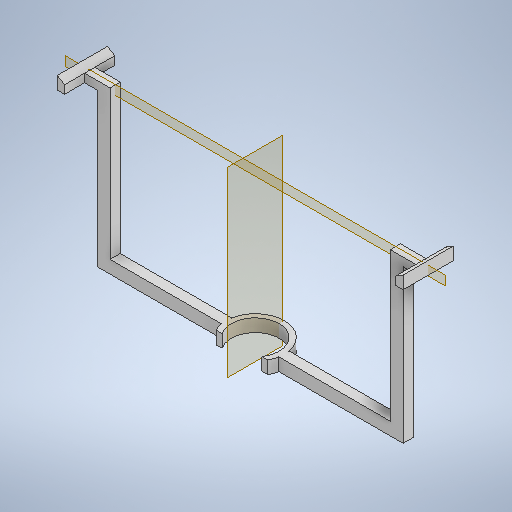
# Autodesk Inventor part: 2025_07_28_Holder_H2_O2_reactor_BOLA_GL14_V0.3
Saved by Autodesk Inventor 2025.1 (Build 291241000, 241)
## iProperties
Created: 2024-08-23
Part Number: 2025_07_28_Holder_H2_O2_reactor_BOLA_GL14_V0.3
Material: Generisch
Document SubType Name: Modeling
Designer: to86hug
Density: 1 g/cm^3
Appearance: Vorgabe
Author: to86hug
Autodesk Inventor part; units mm, degrees
ref_plane "YZ Plane" through (0, 0, 0) normal (1, 0, 0) x (0, 1, 0)
ref_plane "XZ Plane" through (0, 0, 0) normal (0, 1, 0) x (-1, 0, 0)
ref_plane "XY Plane" through (0, 0, 0) normal (0, 0, 1) x (1, 0, 0)
sketch "Skizze1" plane through (0, 0, 0) normal (0, 0, 1) x (1, 0, 0)
  line L0 (-68.016, 1.808) -> (67.584, 1.808)
  line L1 (67.584, 1.808) -> (67.584, -2.192)
  line L2 (67.584, -2.192) -> (-68.016, -2.192)
  line L3 (-68.016, -2.192) -> (-68.016, 1.808)
  line L4 (-68.016, 1.808) -> (67.584, -2.192) construction
  line L5 (67.584, 1.808) -> (-68.016, -2.192) construction
  point P0 (0, 0)
  point P1 (-0.216, -0.192)
  point P2 (-0.216, -0.192)
  dimension "d0" = 135.6
  dimension "d1" = 4
  constraints: 12 end point, 2 midpoint, 2 parallel, 1 horizontal, 1 perpendicular
  measures "d0" distance of L0.start L0.end
  measures "d1" distance of L0.end L1.end
extrude "Extrusion1" add sketch "Skizze1" along normal mid plane 3.25
ref_plane "Arbeitsebene1" through (-68.016, -0.192, 1.625) normal (0, -1, 0) x (1, 0, 0)
sketch "Skizze2" plane through (-68.016, -0.192, 1.625) normal (0, -1, 0) x (1, 0, 0)
  line L0 (0, -3.25) -> (0, 0) projected
  line L1 (0, -3.25) -> (135.6, -3.25) projected
  line L2 (0, 0) -> (2.85, 0)
  line L3 (2.85, 0) -> (2.85, -3.25)
  line L4 (2.85, -3.25) -> (0, -3.25)
  line L5 (0, -3.25) -> (0, 0)
  line L6 (0, 0) -> (0, 1.75)
  line L7 (0, 1.75) -> (2.85, 0)
  line L8 (135.6, -3.25) -> (135.6, 0) projected
  line L9 (135.6, 0) -> (132.75, 0)
  line L10 (132.75, 0) -> (132.75, -3.25)
  line L11 (132.75, -3.25) -> (135.6, -3.25)
  line L12 (135.6, -3.25) -> (135.6, 0)
  line L13 (135.6, 0) -> (135.6, 1.75)
  line L14 (135.6, 1.75) -> (132.75, 0)
  point P0 (68.016, -1.625)
  dimension "d4" = 2.85
  dimension "d5" = 1.75
  dimension "d6" = 2.85
  constraints: 24 end point, 4 parallel, 2 horizontal, 2 perpendicular, 2 point on line, 2 vertical
  measures "d4" distance of L3.end L4.end
  measures "d5" distance of L0.end L6.end
  measures "d6" distance of L11.end L10.end
extrude "Extrusion2" add sketch "Skizze2" along normal mid plane 19.7
sketch "Skizze7" plane through (0, 0, 1.625) normal (0, 0, 1) x (1, 0, 0)
  line L0 (64.734, -2.192) -> (-65.166, -2.192) projected
  line L1 (64.734, 1.808) -> (-65.166, 1.808) projected
  line L2 (64.734, -2.192) -> (59.734, -2.192)
  line L3 (59.734, -2.192) -> (59.734, 1.808)
  line L4 (59.734, 1.808) -> (64.734, 1.808)
  line L5 (64.734, 1.808) -> (64.734, -2.192)
  line L6 (-65.166, -2.192) -> (-65.166, -10.042) projected
  line L7 (-65.166, -2.192) -> (-60.166, -2.192)
  line L8 (-60.166, -2.192) -> (-60.166, 1.808)
  line L9 (-60.166, 1.808) -> (-65.166, 1.808)
  line L10 (-65.166, 1.808) -> (-65.166, -2.192)
  line L11 (59.734, 1.808) -> (-60.166, 1.808)
  line L12 (-60.166, 1.808) -> (-60.166, -2.192)
  line L13 (-60.166, -2.192) -> (59.734, -2.192)
  line L14 (59.734, -2.192) -> (59.734, 1.808)
  point P0 (0, 0)
  point P1 (-60.166, 1.808)
  dimension "d27" = 5
  dimension "d28" = 5
  constraints: 24 end point, 6 parallel, 3 horizontal, 3 perpendicular, 2 point on line
  measures "d27" distance of L3.end L4.end
  measures "d28" distance of L9.end L8.end
extrude "Extrusion7" add sketch "Skizze7" against normal blind 63.25 contours L0 L8 L1 L3
sketch "Skizze8" plane through (-65.166, -2.192, 1.625) normal (0, -1, 0) x (1, 0, 0)
  line L0 (124.9, -3.25) -> (124.9, -63.25) projected
  line L1 (129.9, 0) -> (0, 0) projected
  line L2 (124.9, -3.25) -> (119.9, -3.25)
  line L3 (119.9, -3.25) -> (119.9, 0)
  line L4 (119.9, 0) -> (124.9, 0)
  line L5 (124.9, 0) -> (124.9, -3.25)
  line L6 (4.9878, -3.25) -> (9.9878, -3.25)
  line L7 (9.9878, -3.25) -> (9.9878, 0)
  line L8 (9.9878, 0) -> (4.9878, 0)
  line L9 (4.9878, 0) -> (4.9878, -3.25)
  line L10 (119.9, 0) -> (9.9878, 0)
  line L11 (9.9878, 0) -> (9.9878, -58.25)
  line L12 (9.9878, -58.25) -> (119.9, -58.25)
  line L13 (119.9, -58.25) -> (119.9, 0)
  point P0 (65.166, -1.625)
  dimension "d31" = 5
  dimension "d32" = 5
  dimension "d34" = 58.25
  constraints: 24 end point, 6 parallel, 3 horizontal, 3 perpendicular, 3 point on line
  measures "d31" distance of L3.end L4.end
  measures "d32" distance of L8.end L7.end
  measures "d34" distance of L10.end L11.end
extrude "Extrusion8" cut sketch "Skizze8" against normal through all contours L3 L13 L12 L11 L7 L1
ref_plane "Arbeitsebene2" through (-0.222, -2.192, 1.625) normal (1, 0, 0) x (0, 0, -1)
sketch "Skizze9" plane through (-55.1781, -2.192, -56.625) normal (0, 0, 1) x (1, 0, 0)
  circle A0 centre (54.9561, 2.0001) radius 10.8
  point P0 (55.1781, 2.192)
  dimension "d38" = 21.6
  constraints: 1 centre point
  measures "d38" diameter of A0
extrude "Extrusion9" cut sketch "Skizze9" against normal through all
sketch "Skizze10" plane through (-55.1781, -2.192, -56.625) normal (0, 0, 1) x (1, 0, 0)
  circle A0 centre (54.956, 1.9999) radius 9.4
  circle A1 centre (54.956, 1.9999) radius 11.4
  line L0 (39.8004, -3.1984) -> (71.2174, -3.1984)
  point P0 (55.1781, 2.192)
  point P1 (62.7878, -3.1984)
  point P2 (65.1018, -3.1984)
  point P3 (44.8102, -3.1984)
  point P4 (47.1242, -3.1984)
  dimension "d41" = 18.8
  dimension "d42" = 22.8
  constraints: 2 centre point, 2 end point, 1 coincident, 1 horizontal
  measures "d41" diameter of A0
  measures "d42" diameter of A1
extrude "Extrusion10" add sketch "Skizze10" against normal blind 5 contours A0 L0 A1 picked at (65.5795, 2.9069)
